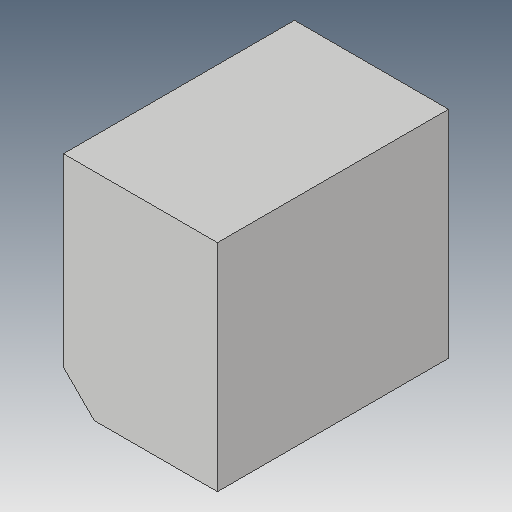
# Autodesk Inventor part: _WT_Aufnahme_Antriebseinheit2
Saved by Autodesk Inventor 2019 (Build 230136000, 136)
## iProperties
Created: 2025-05-01
Part Number: _WT_Aufnahme_Antriebseinheit2
Material: Generisch
Document SubType Name: Modeling
Designer: RP
Density: 1 g/cm^3
Appearance: Vorgabe
Author: RP
Autodesk Inventor part; units mm, degrees
ref_plane "YZ Plane" through (0, 0, 0) normal (1, 0, 0) x (0, 1, 0)
ref_plane "XZ Plane" through (0, 0, 0) normal (0, 1, 0) x (-1, 0, 0)
ref_plane "XY Plane" through (0, 0, 0) normal (0, 0, 1) x (1, 0, 0)
sketch "Skizze1" plane through (0, 0, 0) normal (0, 0, 1) x (1, 0, 0)
  line L0 (26.2311, -43.9228) -> (26.2311, -19.9228)
  line L1 (26.2311, -19.9228) -> (46.2311, -19.9228)
  line L2 (46.2311, -19.9228) -> (46.2311, -47.9228)
  line L3 (46.2311, -47.9228) -> (30.2311, -47.9228)
  line L4 (30.2311, -47.9228) -> (26.2311, -43.9228)
  point P0 (0, 0)
  dimension "d0" = 45
  dimension "d1" = 4
  dimension "d2" = 20
  dimension "d4" = 28
  constraints: 10 end point, 3 perpendicular, 1 vertical
  measures "d0" angle of L4 L0
  measures "d1" horizontal distance of L3.end L0.start
  measures "d2" distance of L0.end L1.end
  measures "d4" distance of L1.end L2.end
extrude "Extrusion1" add sketch "Skizze1" along normal mid plane 30
